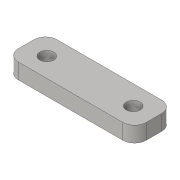
# Autodesk Inventor part: 9 peristaltic pump clamp
Saved by Autodesk Inventor 2016 (Build 200138000, 138)
## iProperties
Created: 2018-08-21
Part Number: 9 peristaltic pump clamp
Material: Generic
Document SubType Name: Modeling
Designer: mrbeh
Density: 1 g/cm^3
Appearance: Default
Author: mrbeh
Autodesk Inventor part; units mm, degrees
ref_plane "YZ Plane" through (0, 0, 0) normal (1, 0, 0) x (0, 1, 0)
ref_plane "XZ Plane" through (0, 0, 0) normal (0, 1, 0) x (-1, 0, 0)
sketch "Sketch1" plane through (0, 0, 0) normal (0, 1, 0) x (-1, 0, 0)
  line L0 (0, 0) -> (33, 0)
  line L1 (33, 0) -> (33, -10)
  line L2 (33, -10) -> (0, -10)
  line L3 (0, -10) -> (0, 0)
  dimension "d0" = 33
  dimension "d1" = 10
  constraints: 8 end point, 2 parallel, 1 horizontal, 1 perpendicular
  measures "d0" distance of L1.end L2.end
  measures "d1" distance of L0.end L1.end
extrude "Extrusion1" add sketch "Sketch1" along normal blind 4
sketch "Sketch2" plane through (0, 4, 0) normal (0, 1, 0) x (1, 0, 0)
  circle A0 centre (-5.343, 5) radius 1.8
  point P0 (0, 0)
  dimension "d9" = 3.6
  constraints: 1 centre point
  measures "d9" diameter of A0
extrude "Extrusion2" cut sketch "Sketch2" against normal blind 4
ref_plane "Work Plane1" through (-16.5, 0, 0) normal (1, 0, 0) x (0, 0, -1)
mirror "Mirror1" about plane through (-16.5, 0, 0) normal (1, 0, 0) of "Extrusion2"
fillet "Fillet1" radius 3 4 edges at (-33, 2, 0) (-33, 2, -10) (0, 2, 0) (0, 2, -10)
body "Solid1"
